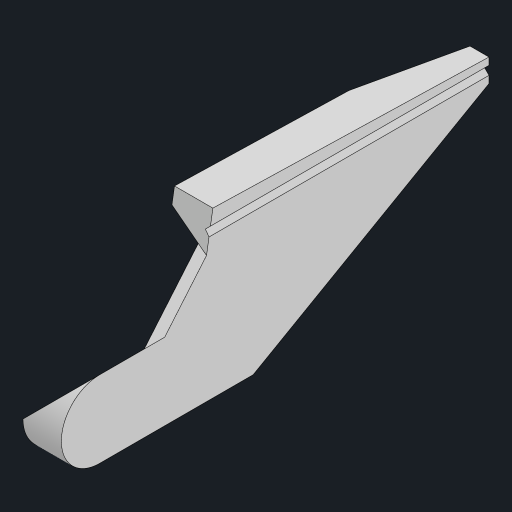
# Autodesk Inventor part: om_Body_R
Saved by Autodesk Inventor 2023 (Build 270158000, 158)
## iProperties
Created: 2022-06-16
Part Number: om_Body_R
Material: 一般
Document SubType Name: Modeling
Designer: legot
Density: 1 g/cm^3
Appearance: 既定
Author: legot
Autodesk Inventor part; units mm, degrees
ref_plane "YZ Plane" through (0, 0, 0) normal (1, 0, 0) x (0, 1, 0)
ref_plane "XZ Plane" through (0, 0, 0) normal (0, 1, 0) x (-1, 0, 0)
ref_plane "XY Plane" through (0, 0, 0) normal (0, 0, 1) x (1, 0, 0)
sketch "スケッチ1" plane through (0, 0, 0) normal (1, 0, 0) x (0, 1, 0)
  line L0 (-24.6571, 4.1262) -> (-57.1587, 31.3982)
  line L1 (-57.1587, 31.3982) -> (-57.1587, 98.7205)
  arc A0 (-82.1587, 98.7205) -> (-107.1587, 73.7205) centre (-82.1587, 73.7205) ccw
  line L2 (-107.1587, 73.7205) -> (-107.1587, -26.2795)
  line L3 (-107.1587, -26.2795) -> (-19.7119, -179.9383)
  line L4 (-19.7119, -179.9383) -> (-4.7119, -179.9383)
  line L5 (-4.7119, -179.9383) -> (0, 0)
  line L6 (0, 0) -> (0, -120.6859) construction
  line L7 (-24.6571, 4.1262) -> (0, 0)
  line L8 (0, 0) -> (23.9477, 0) construction
  line L9 (0.4951, 2.9589) -> (49.8094, -5.2935)
  line L10 (49.8094, -5.2935) -> (49.3143, -8.2524)
  line L11 (49.3143, -8.2524) -> (0, 0)
  line L12 (37.4809, -3.2304) -> (41.607, 21.4267)
  line L13 (130.3727, 6.5724) -> (-47.1587, 36.281)
  line L14 (-57.1587, 98.7205) -> (-82.1587, 98.7205)
  line L15 (-82.1587, 98.7205) -> (-82.1587, 19.7405)
  line L16 (-82.1587, 19.7405) -> (-37.35, -17.8584)
  line L17 (-37.35, -17.8584) -> (-24.6571, 4.1262)
  line L18 (-57.1587, 31.3982) -> (-82.1587, 19.7405)
  line L19 (0, 0) -> (0.4951, 2.9589)
  point P0 (-99.8363, 91.3982)
  dimension "d0" = 1.5
  dimension "d1" = 25
  dimension "d2" = 25
  dimension "d3" = 130
  dimension "d4" = 9.5
  dimension "d5" = 60
  dimension "d7" = 3
  dimension "d9" = 50
  dimension "d11" = 100
  dimension "d12" = 180
  dimension "d13" = 25
  dimension "d14" = 10
  dimension "d15" = 180
  dimension "d16" = 15
  dimension "d19" = 50
  dimension "d34" = 25
  dimension "d35" = 80
  dimension "d36" = 65
  dimension "d54" = 12.5
  constraints: 40 end point, 5 perpendicular, 4 vertical, 3 point on circle, 2 horizontal, 2 parallel, 2 tangent, 1 centre point, 1 collinear, 1 midpoint, 1 point on line
  measures "d0" angle of L6 L5
  measures "d1" distance of L5.end L0.start
  measures "d2" radius of A0
  measures "d3" angle of L6 L0
  measures "d4" angle of L8 L7
  measures "d5" vertical distance of point (-99.836, 91.398) L0.end
  measures "d7" distance of L9.end L10.end
  measures "d9" distance of L9.start L9.end
  measures "d11" distance of L2.start L2.end
  measures "d12" distance of L13.start L13.end
  measures "d13" distance of L12.start L12.end
  measures "d14" distance from line of L13.end L1
  measures "d15" distance of L4.end L5.end
  measures "d16" distance of L3.end L4.end
  measures "d19" distance between parallel lines of L1 L2
  measures "d34" distance between parallel lines of L0 L16
  measures "d35" angle of L17 L16
  measures "d36" angle of L18 L15
  measures "d54" distance from line of L10.end L12
extrude "押し出し1" add sketch "スケッチ1" along normal mid plane 50 contours L7 L5 L4 L3 L2 A0 L15 L16 L17
ref_plane "作業平面1" through (0, -82.1587, 98.7205) normal (0, 0, 1) x (1, 0, 0)
ref_plane "作業平面3" through (0, -82.1587, 19.7405) normal (0, -0.7660444, 0.6427876) x (1, 0, 0)
sketch "スケッチ5" plane through (0, -82.1587, 19.7405) normal (0, -0.7660444, 0.6427876) x (1, 0, 0)
  line L0 (-25, 0) -> (0, 25)
  line L1 (25, 0) -> (-25, 0)
  line L2 (0, 25) -> (25, 0)
  point P0 (0, 37.6885)
  constraints: 6 end point, 1 coincident, 1 horizontal
extrude "押し出し5" add sketch "スケッチ5" against normal up to surface surface through (0, -24.6571, 4.1262) normal (0, -0.8660254, 0.5)
sketch "スケッチ6" plane through (0, -82.1587, 98.7205) normal (0, 0, 1) x (1, 0, 0)
  line L0 (-25, 0) -> (25, 0) projected
  line L1 (-25, 0) -> (0, 25)
  line L2 (0, 25) -> (25, 0)
  line L3 (25, 0) -> (-25, 0)
  point P0 (0, 82.1587)
  constraints: 6 end point, 1 collinear, 1 perpendicular
extrude "押し出し6" add sketch "スケッチ6" against normal through all
sketch "スケッチ7" plane through (-25, 0, 0) normal (0, 0.1650476, 0.9862856) x (1, 0, 0)
  line L0 (50, -25) -> (25, -25) projected
  line L1 (50, 0) -> (50, -25) projected
  line L2 (0, 0) -> (50, 0) projected
  line L3 (0, -25) -> (0, 0) projected
  line L4 (25, -25) -> (0, -25) projected
  line L5 (25, -25) -> (50, -10)
  line L6 (50, 10.2569) -> (50, 0) projected
  line L7 (25, -25) -> (0, -10)
  point P0 (25, 0)
  dimension "d41" = 10
  constraints: 4 end point, 2 point on line, 1 horizontal alignment
  measures "d41" distance from line of L2 L5.end
ref_plane "作業平面4" through (-2.3477, -23.4652, 6.1907) normal (0.3897863, -0.5330063, 0.75098) x (0.7016738, -0.3562491, -0.6170416)
sketch "スケッチ8" plane through (-2.3477, -23.4652, 6.1907) normal (0.3897863, -0.5330063, 0.75098) x (0.7016738, -0.3562491, -0.6170416)
  line L0 (3.3458, 0) -> (38.9749, 0) projected
  line L1 (3.3458, 0) -> (17.1448, 25.6824) projected
  line L2 (20.8877, 14.9106) -> (38.9749, 0) projected
  line L3 (38.9749, 0) -> (17.1448, 25.6824)
  point P0 (-2.8922, 17.9531)
  constraints: 2 end point
extrude "押し出し7" cut sketch "スケッチ8" along normal blind 10
ref_plane "作業平面5" through (-9.961, -29.7145, -4.6333) normal (-0.3897863, -0.5330063, 0.75098) x (0.7016738, 0.3562491, 0.6170416)
sketch "スケッチ9" plane through (-9.961, -29.7145, -4.6333) normal (-0.3897863, -0.5330063, 0.75098) x (0.7016738, 0.3562491, 0.6170416)
  line L0 (14.196, 0) -> (0.397, 25.6824) projected
  line L1 (-21.4331, 0) -> (14.196, 0) projected
  line L2 (-21.4331, 0) -> (-3.3458, 14.9106) projected
  line L3 (-21.4331, 0) -> (0.397, 25.6824)
  point P0 (20.4341, 17.9531)
  constraints: 2 end point
extrude "押し出し8" cut sketch "スケッチ9" along normal blind 10
sketch "スケッチ10" plane through (0, 0, 0) normal (1, 0, 0) x (0, 1, 0)
  arc A0 (-82.1587, 98.7205) -> (-107.1587, 73.7205) centre (-82.1587, 73.7205) ccw projected
  arc A1 (-82.1587, 98.7205) -> (-107.1587, 73.7205) centre (-82.1587, 73.7205) ccw projected
  circle A2 centre (-82.1587, 73.7205) radius 25
  line L0 (-82.1587, 19.7405) -> (-57.1587, 31.3982) projected
  line L1 (-82.1587, 98.7205) -> (-82.1587, 19.7405) projected
  line L2 (-57.1587, 98.7205) -> (-82.1587, 98.7205) projected
  line L3 (-57.1587, 98.7205) -> (-57.1587, 31.3982) projected
  point P0 (0, 0)
  point P1 (-57.1587, 73.7205)
  constraints: 1 centre point, 1 coincident, 1 concentric
extrude "押し出し9" cut sketch "スケッチ10" along normal through all both and the other way through all contours L2 L3 A2
ref_plane "作業平面6" through (25, -107.1587, -26.2795) normal (0, -0.7660444, 0.6427876) x (1, 0, 0)
sketch "スケッチ11" plane through (25, -107.1587, -26.2795) normal (0, -0.7660444, 0.6427876) x (1, 0, 0)
  line L0 (-50, -61.4998) -> (0, -61.4998) projected
  line L1 (0, 0) -> (-15, -61.4998)
  line L2 (-35, -61.4998) -> (-50, 0)
  line L3 (-35, -61.4998) -> (-15, -61.4998)
  line L4 (0, 0) -> (0, -61.4998) projected
  line L5 (-50, -61.4998) -> (-50, 0) projected
  point P0 (-25, 89.0115)
  point P1 (-25, -61.4998)
  dimension "d48" = 20
  constraints: 6 end point, 2 coincident, 2 midpoint, 2 point on line, 1 collinear, 1 equal length
  measures "d48" distance of L1.end L2.start
extrude "押し出し10" cut sketch "スケッチ11" against normal through all
sketch "スケッチ12" plane through (12.3517, -4.7119, -179.9383) normal (0, 0, -1) x (-1, 0, 0)
  line L0 (22.3517, -15) -> (24.7033, 0) projected
  line L1 (12.3517, -4.6716) -> (9.5232, -7.5)
  line L2 (9.5232, -7.5) -> (12.3517, -10.3284)
  line L3 (12.3517, -10.3284) -> (15.1801, -7.5)
  line L4 (15.1801, -7.5) -> (12.3517, -4.6716)
  point P0 (12.3517, 4.7119)
  point P1 (23.5275, -7.5)
  dimension "d51" = 4
  constraints: 8 end point, 2 parallel, 2 perpendicular, 2 vertical alignment, 1 horizontal alignment, 1 midpoint
  measures "d51" distance of L2.end L3.end
extrude "押し出し11" cut sketch "スケッチ12" against normal through all
sketch "スケッチ13" plane through (0, 0, 0) normal (1, 0, 0) x (0, 1, 0)
  line L0 (30.6642, 121.32) -> (-119.0398, 121.32)
  line L1 (-119.0398, 121.32) -> (-119.0398, -193.8132)
  line L2 (-119.0398, -193.8132) -> (30.6642, -193.8132)
  line L3 (30.6642, -193.8132) -> (30.6642, 121.32)
  point P0 (0, 0)
  constraints: 8 end point, 2 parallel, 1 horizontal, 1 perpendicular
extrude "押し出し12" cut sketch "スケッチ13" along normal through all
